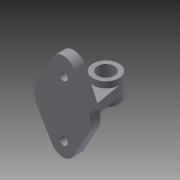
# Autodesk Inventor part: HW 6 Part 2
Saved by Autodesk Inventor 2015 SP1 (Build 190203100, 203)
## iProperties
Created: 2016-02-10
Part Number: HW 6 Part 2
Material: Generic
Document SubType Name: Modeling
Designer: melissa.roth
Density: 1 g/cm^3
Appearance: Default
Author: melissa.roth
Autodesk Inventor part; units mm, degrees
ref_plane "YZ Plane" through (0, 0, 0) normal (1, 0, 0) x (0, 1, 0)
ref_plane "XZ Plane" through (0, 0, 0) normal (0, 1, 0) x (-1, 0, 0)
ref_plane "XY Plane" through (0, 0, 0) normal (0, 0, 1) x (1, 0, 0)
sketch "Sketch1" plane through (0, 0, 0) normal (0, 0, 1) x (1, 0, 0)
  arc A0 (22.6557, 3.9649) -> (-22.6557, 3.9649) centre (0, 0) ccw
  line L0 (-33.5, -58) -> (33.5, -58)
  line L1 (0, -58) -> (0, -55)
  line L2 (-33.5, -58) -> (-22.6557, 3.9649)
  line L3 (33.5, -58) -> (22.6557, 3.9649)
  circle A1 centre (0, 0) radius 15
  dimension "d0" = 46
  dimension "d1" = 67
  dimension "d2" = 58
  dimension "d3" = 0
  dimension "d4" = 30
  constraints: 8 end point, 2 centre point, 2 coincident, 2 point on circle, 2 tangent, 1 horizontal, 1 midpoint, 1 vertical
  measures "d0" diameter of A0
  measures "d1" distance of L0.start L0.end
  measures "d2" distance from line of L0 A0.centre
  measures "d3" horizontal distance of L1.start point (0, 0)
  measures "d4" diameter of A1
extrude "Extrusion1" add sketch "Sketch1" along normal blind 18
sketch "Sketch2" plane through (0, 0, 18) normal (0, 0, 1) x (1, 0, 0)
  circle A0 centre (0, 0) radius 23
  circle A1 centre (0, 0) radius 15
  dimension "d7" = 46
  dimension "d8" = 30
  constraints: 2 centre point, 2 coincident
  measures "d7" diameter of A0
  measures "d8" diameter of A1
extrude "Extrusion2" add sketch "Sketch2" along normal blind 11
sketch "Sketch3" plane through (0, 0, 0) normal (0, 0, -1) x (-1, 0, 0)
  circle A0 centre (0, 0) radius 23
  circle A1 centre (0, 0) radius 15
  dimension "d11" = 46
  dimension "d12" = 30
  constraints: 2 centre point, 2 coincident
  measures "d11" diameter of A0
  measures "d12" diameter of A1
extrude "Extrusion3" add sketch "Sketch3" along normal blind 11
sketch "Sketch4" plane through (-33.5, -58, 0) normal (0, -1, 0) x (1, 0, 0)
  circle A0 centre (33.5, 59) radius 7.5
  circle A1 centre (33.5, -41) radius 7.5
  line L0 (0, 0) -> (0, 18) projected
  line L1 (14.2497, 79.1265) -> (-13.8345, 28.3639)
  line L2 (-13.2531, -11.3795) -> (13.4134, -56.4168)
  line L3 (51.5943, -55.8582) -> (76.7638, -10.3639)
  line L4 (77.9107, 26.1277) -> (53.3811, 77.8966)
  arc A2 (53.3811, 77.8966) -> (14.2497, 79.1265) centre (33.5, 68.4764) ccw
  arc A3 (76.7638, -10.3639) -> (77.9107, 26.1277) centre (41.7632, 9) ccw
  arc A4 (-13.8345, 28.3639) -> (-13.2531, -11.3795) centre (21.1661, 9) ccw
  arc A5 (13.4134, -56.4168) -> (51.5943, -55.8582) centre (32.344, -45.2081) ccw
  line L5 (10.5, 18) -> (56.5, 18) projected
  line L6 (33.5, 18) -> (33.5, 0)
  line L7 (67, 0) -> (67, 18) projected
  line L8 (67, 9) -> (0, 9)
  line L9 (41.7632, 9) -> (21.1661, 9)
  point P0 (56.1557, 18)
  point P1 (10.8443, 18)
  dimension "d15" = 15
  dimension "d16" = 15
  dimension "d17" = 100
  dimension "d19" = 22
  dimension "d21" = 40
  dimension "d24" = 40
  dimension "d25" = 0
  dimension "d26" = 22
  dimension "d28" = 0
  dimension "d29" = 0
  constraints: 14 end point, 8 point on circle, 8 tangent, 6 centre point, 3 midpoint, 1 parallel, 1 vertical
  measures "d15" diameter of A0
  measures "d16" diameter of A1
  measures "d17" distance of A1.centre A0.centre
  measures "d19" radius of A2
  measures "d21" radius of A3
  measures "d24" radius of A4
  measures "d25" vertical distance of L9.end L9.start
  measures "d26" radius of A5
  measures "d28" distance from line of L8 L9.start
  measures "d29" distance from line of A2.centre L6
extrude "Extrusion4" add sketch "Sketch4" along normal blind 18
body "Solid1"
